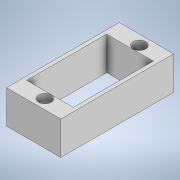
# Autodesk Inventor part: servo housing electric boogaloo
Saved by Autodesk Inventor 2022 (Build 260153000, 153)
## iProperties
Created: 2022-02-04
Part Number: servo housing electric boogaloo
Material: Generic
Document SubType Name: Modeling
Designer: cyber
Density: 1 g/cm^3
Appearance: Default
Author: cyber
Autodesk Inventor part; units mm, degrees
ref_plane "YZ Plane" through (0, 0, 0) normal (1, 0, 0) x (0, 1, 0)
ref_plane "XZ Plane" through (0, 0, 0) normal (0, 1, 0) x (-1, 0, 0)
ref_plane "XY Plane" through (0, 0, 0) normal (0, 0, 1) x (1, 0, 0)
sketch "Sketch2" plane through (0, 0, 0) normal (0, 1, 0) x (-1, 0, 0)
  line L0 (8.14, 16.9) -> (-8.14, 16.9)
  line L1 (-8.14, 16.9) -> (-8.14, -16.9)
  line L2 (-8.14, -16.9) -> (8.14, -16.9)
  line L3 (8.14, -16.9) -> (8.14, 16.9)
  line L4 (8.14, 16.9) -> (-8.14, -16.9) construction
  line L5 (-8.14, 16.9) -> (8.14, -16.9) construction
  point P0 (0, 0)
  dimension "d0" = 33.8
  dimension "d1" = 16.28
  constraints: 12 end point, 2 midpoint, 2 parallel, 1 horizontal, 1 perpendicular
  measures "d0" distance of L2.end L0.start
  measures "d1" distance of L1.end L2.end
sketch "Sketch3" plane through (0, 0, 0) normal (0, 1, 0) x (-1, 0, 0)
  line L0 (-7, -12) -> (7, -12)
  line L1 (7, -12) -> (7, 12)
  line L2 (7, 12) -> (-7, 12)
  line L3 (-7, 12) -> (-7, -12)
  line L4 (-7, -12) -> (7, 12) construction
  line L5 (7, -12) -> (-7, 12) construction
  point P0 (0, 0)
  dimension "d2" = 24
  dimension "d3" = 14
  constraints: 12 end point, 2 midpoint, 2 parallel, 1 horizontal, 1 perpendicular
  measures "d2" distance of L0.end L1.end
  measures "d3" distance of L1.end L2.end
extrude "Extrusion1" add sketch "Sketch2" along normal blind 10
extrude "Extrusion2" cut sketch "Sketch3" along normal blind 10
sketch "Sketch5" plane through (0, 10, 0) normal (0, 1, 0) x (1, 0, 0)
  line L0 (7, -12) -> (-7, -12) projected
  point P0 (0, 0)
  point P1 (0.476, -14)
  dimension "d22" = 2
  measures "d22" distance from line of L0 point (0.476, -14)
hole "Hole1" at (0.476, 10, 14) direction (0, -1, 0) diameter 3.81 depth 10
sketch "Sketch6" plane through (0, 10, 0) normal (0, 1, 0) x (1, 0, 0)
  line L0 (7, 12) -> (-7, 12) projected
  point P0 (0, 0)
  point P1 (0.8061, 14)
  dimension "d30" = 2
  measures "d30" distance from line of L0 point (0.806, 14)
hole "Hole2" at (0.8061, 10, -14) direction (0, -1, 0) diameter 3.81 depth 10
body "Solid1"
